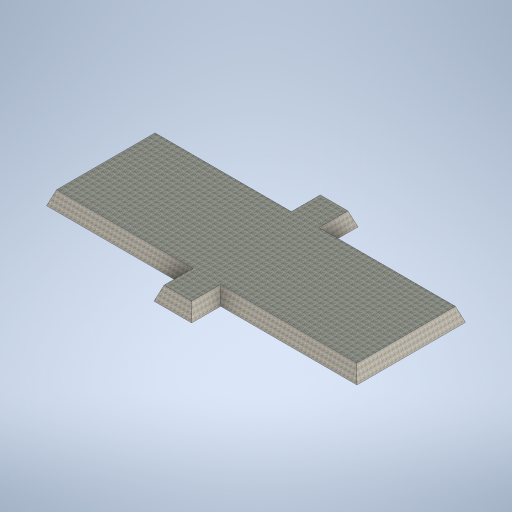
# Autodesk Inventor part: main_floor
Saved by Autodesk Inventor 2024.2 (Build 282272000, 272)
## iProperties
Created: 2024-05-24
Part Number: main_floor
Material: Limestone
Document SubType Name: Modeling
Designer: LOSTER_1
Density: 2.6 g/cm^3
Appearance: Limestone - Ashlar Coursed
Author: LOSTER_1
Autodesk Inventor part; units mm, degrees
ref_plane "YZ Plane" through (0, 0, 0) normal (1, 0, 0) x (0, 1, 0)
ref_plane "XZ Plane" through (0, 0, 0) normal (0, 1, 0) x (-1, 0, 0)
ref_plane "XY Plane" through (0, 0, 0) normal (0, 0, 1) x (1, 0, 0)
sketch "Sketch1" plane through (0, 0, 0) normal (0, 1, 0) x (-1, 0, 0)
  line L0 (-18589.1353, 7057.2083) -> (-18589.1353, -7090.0785)
  line L1 (18609.9901, -7090.0785) -> (18609.9901, 7057.2083)
  line L2 (18609.9901, 7057.2083) -> (21609.9901, 7057.2083)
  line L3 (21609.9901, 7057.2083) -> (21609.9901, -7090.0785)
  line L4 (21609.9901, -7090.0785) -> (18609.9901, -7090.0785)
  line L5 (18609.9901, -7090.0785) -> (18609.9901, 7057.2083)
  line L6 (-18589.1353, 7057.2083) -> (-21589.1353, 7057.2083)
  line L7 (-21589.1353, 7057.2083) -> (-21589.1353, -7090.0785)
  line L8 (-21589.1353, -7090.0785) -> (-18589.1353, -7090.0785)
  line L9 (-18589.1353, -7090.0785) -> (-18589.1353, 7057.2083)
  line L10 (1994.5778, 9218.7168) -> (-1973.723, 9218.7168)
  line L11 (-1973.723, -9251.4689) -> (1994.5778, -9251.4689)
  line L12 (1994.5778, -9251.4689) -> (1994.5778, -7090.0785)
  line L13 (1994.5778, 7057.2083) -> (1994.5778, 9218.7168)
  line L14 (18609.9901, 7057.2083) -> (1994.5778, 7057.2083)
  line L15 (-1973.723, 7057.2083) -> (-18589.1353, 7057.2083)
  line L16 (-1973.723, 9218.7168) -> (-1973.723, 7057.2083)
  line L17 (-1973.723, -7090.0785) -> (-1973.723, -9251.4689)
  line L18 (-18589.1353, -7090.0785) -> (-1973.723, -7090.0785)
  line L19 (1994.5778, -7090.0785) -> (18609.9901, -7090.0785)
  line L20 (1994.5778, 9218.7168) -> (-1973.723, 9218.7168)
  line L21 (-1973.723, 9218.7168) -> (-1973.723, 11218.7168)
  line L22 (-1973.723, 11218.7168) -> (1994.5778, 11218.7168)
  line L23 (1994.5778, 11218.7168) -> (1994.5778, 9218.7168)
  line L24 (1994.5778, -9251.4689) -> (-1973.723, -9251.4689)
  line L25 (-1973.723, -9251.4689) -> (-1973.723, -11251.4689)
  line L26 (-1973.723, -11251.4689) -> (1994.5778, -11251.4689)
  line L27 (1994.5778, -11251.4689) -> (1994.5778, -9251.4689)
  point P0 (-1973.723, 9218.7168)
  point P1 (1994.5778, -9251.4689)
  dimension "d0" = 3000
  dimension "d1" = 3000
  dimension "d2" = 2000
  dimension "d3" = 2000
  constraints: 56 end point, 18 parallel, 8 perpendicular, 7 horizontal, 2 point on line
  measures "d0" distance of L3.end L4.end
  measures "d1" distance of L8.end L7.end
  measures "d2" distance of L20.end L21.end
  measures "d3" distance of L25.end L24.end
extrude "Extrusion1" add sketch "Sketch1" against normal blind 2000 draft 20
body "Solid1"
